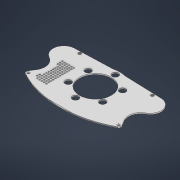
# Autodesk Inventor part: buttonMount-backingPlate
Saved by Autodesk Inventor 2022 (Build 260153000, 153)
## iProperties
Created: 2022-07-18
Part Number: buttonMount-backingPlate
Material: Generic
Document SubType Name: Modeling
Designer: matti
Density: 1 g/cm^3
Appearance: Default
Author: matti
Autodesk Inventor part; units mm, degrees
ref_plane "YZ Plane" through (0, 0, 0) normal (1, 0, 0) x (0, 1, 0)
ref_plane "XZ Plane" through (0, 0, 0) normal (0, 1, 0) x (-1, 0, 0)
ref_plane "XY Plane" through (0, 0, 0) normal (0, 0, 1) x (1, 0, 0)
sketch "Sketch1" plane through (0, 0, 0) normal (0, 1, 0) x (-1, 0, 0)
  arc A0 (1.4897, -42.9742) -> (29.2283, -31.5389) centre (0, 0) ccw
  line L0 (1.4897, -42.9742) -> (76.5814, -40.3711)
  arc A1 (76.5814, -40.3711) -> (86.503, -3.4322) centre (75.8885, -20.3831) ccw
  line L1 (86.503, -3.4322) -> (83.9054, -1.8056)
  arc A2 (77.5688, 25.7598) -> (83.9054, -1.8056) centre (94.5198, 15.1453) ccw
  line L2 (77.5688, 25.7598) -> (83.1923, 34.7403)
  arc A3 (83.1923, 34.7403) -> (84.2595, 38.4553) centre (77.2595, 38.4553) ccw
  line L3 (84.2595, 38.4553) -> (84.2595, 38.4997)
  arc A4 (84.2595, 38.4997) -> (81.6444, 42.8943) centre (79.2595, 38.4997) ccw
  arc A5 (81.6444, 42.8943) -> (0, 63) centre (2.3779, -103.1661) ccw
  arc A6 (0, 63) -> (-81.6444, 42.8943) centre (-2.3779, -103.1661) ccw
  arc A7 (-81.6444, 42.8943) -> (-84.2595, 38.4997) centre (-79.2595, 38.4997) ccw
  line L4 (-84.2595, 38.4997) -> (-84.2595, 38.4553)
  arc A8 (-84.2595, 38.4553) -> (-83.1923, 34.7403) centre (-77.2595, 38.4553) ccw
  line L5 (-83.1923, 34.7403) -> (-77.5688, 25.7598)
  arc A9 (-83.9054, -1.8056) -> (-77.5688, 25.7598) centre (-94.5198, 15.1453) ccw
  line L6 (-83.9054, -1.8056) -> (-86.503, -3.4322)
  arc A10 (-86.503, -3.4322) -> (-76.5814, -40.3711) centre (-75.8885, -20.3831) ccw
  line L7 (-76.5814, -40.3711) -> (-1.4897, -42.9742)
  arc A11 (-29.557, -31.2311) -> (-1.4897, -42.9742) centre (0, 0) ccw
  arc A12 (43, 0) -> (-29.557, -31.2311) centre (0, 0) ccw
  arc A13 (29.2283, -31.5389) -> (43, 0) centre (0, 0) ccw
  arc A14 (43, 0) -> (-33.1962, -27.3316) centre (0, 0) ccw
  arc A15 (13.2392, -24.6723) -> (-13.4968, -24.5323) centre (0, 0) ccw
  circle A16 centre (-30.3109, -17.5) radius 5.5
  circle A17 centre (30.3109, -17.5) radius 5.5
  circle A18 centre (30.3109, 17.5) radius 5.5
  circle A19 centre (0, 35) radius 5.5
  circle A20 centre (-30.3109, 17.5) radius 5.5
  circle A21 centre (0, -35) radius 5.5
  arc A22 (-13.4968, -24.5323) -> (13.2392, -24.6723) centre (0, 0) ccw
  arc A23 (-29.557, -31.2311) -> (-1.4897, -42.9742) centre (0, 0) ccw
  arc A24 (-1.4897, -42.9742) -> (1.4897, -42.9742) centre (0, 0) ccw
  arc A25 (1.4897, -42.9742) -> (29.2283, -31.5389) centre (0, 0) ccw
  arc A26 (32.9081, -27.6777) -> (43, 0) centre (0, 0) ccw
  circle A27 centre (79.2595, 38.4997) radius 0.75
  circle A28 centre (63.8182, -36.3301) radius 1.25
  circle A29 centre (79.2595, 38.4997) radius 1.5
  circle A30 centre (63.8182, -36.3301) radius 2
  arc A31 (0, 61.9999) -> (-81.1674, 42.0154) centre (-2.3779, -103.1661) ccw
  arc A32 (81.1674, 42.0154) -> (0, 61.9999) centre (2.3779, -103.1661) ccw
  arc A33 (83.2595, 38.4997) -> (81.1674, 42.0154) centre (79.2595, 38.4997) ccw
  line L8 (83.2595, 38.4997) -> (83.2595, 38.4553)
  arc A34 (82.3448, 35.271) -> (83.2595, 38.4553) centre (77.2595, 38.4553) ccw
  line L9 (82.3448, 35.271) -> (76.7213, 26.2905)
  arc A35 (76.7213, 26.2905) -> (83.3746, -2.6531) centre (94.5198, 15.1453) ccw
  line L10 (83.3746, -2.6531) -> (85.9722, -4.2797)
  arc A36 (76.5468, -39.3717) -> (85.9722, -4.2797) centre (75.8885, -20.3831) ccw
  line L11 (-10.6691, -41.6554) -> (-76.5468, -39.3717)
  arc A37 (-85.9722, -4.2797) -> (-76.5468, -39.3717) centre (-75.8885, -20.3831) ccw
  line L12 (-85.9722, -4.2797) -> (-83.3746, -2.6531)
  arc A38 (-83.3746, -2.6531) -> (-76.7213, 26.2905) centre (-94.5198, 15.1453) ccw
  line L13 (-76.7213, 26.2905) -> (-82.3448, 35.271)
  arc A39 (-83.2595, 38.4553) -> (-82.3448, 35.271) centre (-77.2595, 38.4553) ccw
  line L14 (-83.2595, 38.4553) -> (-83.2595, 38.4997)
  arc A40 (-81.1674, 42.0154) -> (-83.2595, 38.4997) centre (-79.2595, 38.4997) ccw
  line L15 (76.5468, -39.3717) -> (10.6691, -41.6554)
  line L16 (0, 0) -> (0, 12.9729)
  line L17 (0, 0) -> (12.9729, 0) construction
  circle A41 centre (-79.2595, 38.4997) radius 1.5
  circle A42 centre (-79.2595, 38.4997) radius 0.75
  circle A43 centre (-63.8182, -36.3301) radius 2
  circle A44 centre (-63.8182, -36.3301) radius 1.25
  point P0 (-77.2595, 38.4553)
  point P1 (-1.4897, -42.9742)
  dimension "d0" = 1.5
  dimension "d1" = 2.5
  dimension "d3" = 3
  dimension "d4" = 4
  dimension "d6" = 1
  dimension "d7" = 90
  constraints: 65 point on circle, 45 centre point, 36 end point, 6 coincident, 6 symmetric about line, 1 horizontal, 1 perpendicular, 18 other
  measures "d0" diameter of A27
  measures "d1" diameter of A28
  measures "d3" diameter of A29
  measures "d4" diameter of A30
  measures "d6" radial gap between concentric circles of A6 A31
  measures "d7" angle of L17 L16
extrude "Extrusion1" add sketch "Sketch1" along normal blind 2 contours A24 A11 A12 A13 A0 | A0 A13 A12 A11 L11 A37 L12 A38 L13 A39 L14 A40 A31 A32 A33 L8 A34 L9 A35 L10 A36 L15
chamfer "Chamfer1" distance 0.75 angle 45 4 edges at (80.7595, 2, 38.4997) (65.8182, 2, -36.3301) (-61.8182, 2, -36.3301) (-77.7595, 2, 38.4997)
sketch "Sketch2" plane through (0, 2, 0) normal (0, 1, 0) x (1, 0, 0)
  arc A0 (-39.2332, -48.7478) -> (0.0157, -53.5719) centre (-0.7049, 102.6414) ccw
  line L0 (-43, 8.6615) -> (-61.5767, 28.5094)
  line L1 (-72.4279, 0.8961) -> (-72.4279, -43.1434)
  line L2 (-72.4279, -43.1434) -> (-56.6935, -52.2964)
  arc A1 (-61.5767, 28.5094) -> (-82.4964, 5.3099) centre (-75.8885, 20.3831) ccw
  line L3 (-43, 8.6615) -> (-43, -43.9022)
  arc A2 (57.4373, -52.0723) -> (56.4451, -43.938) centre (55.7026, -48.1562) ccw
  arc A3 (-43, -43.9022) -> (-39.2332, -48.7478) centre (-38, -43.9022) ccw
  line L4 (-72.4279, 0.8961) -> (-82.4964, 5.3099)
  arc A4 (-56.6935, -52.2964) -> (57.4373, -52.0723) centre (0.0404, 116.5749) ccw
  arc A5 (0.0157, -53.5719) -> (56.4451, -43.938) centre (-2.1892, 129.4242) ccw
  circle A6 centre (-75.8885, 20.3831) radius 1.1028
  line L5 (-72.4279, -43.1434) -> (-43, -43.1434)
  line L6 (-72.4279, 0.8961) -> (-52.8672, 19.2039)
  line L7 (-43, -43.1434) -> (-47, -43.1434)
  line L8 (-43, -39.1434) -> (-43, -43.1434)
  circle A7 centre (-47, -39.1434) radius 1.25
  line L9 (-72.4279, -43.1434) -> (-68.4279, -43.1434)
  line L10 (-68.4279, -43.1434) -> (-68.4279, -39.1434)
  line L11 (-68.4279, -39.1434) -> (-72.4279, -39.1434)
  line L12 (-72.4279, -39.1434) -> (-72.4279, -43.1434)
  point P0 (0, 0)
  point P1 (0, 0)
  point P2 (-43, -47.7389)
  point P3 (0, -63)
  dimension "d15" = 2.5
  dimension "d16" = 4
  dimension "d17" = 4
  constraints: 26 end point, 13 point on circle, 9 centre point, 3 perpendicular, 3 point on line, 2 horizontal, 2 parallel, 2 tangent
  measures "d15" diameter of A7
  measures "d16" distance of L11.end L10.end
  measures "d17" distance of L10.end L9.end
extrude "Extrusion2" cut sketch "Sketch2" against normal through all contours A7
pattern_linear "Rectangular Pattern1" count 13 spacing 4 along (0, 0, -1) count 6 spacing 4 along (-1, 0, 0) of "Extrusion2"
sketch "Sketch3" plane through (0, 2, 0) normal (0, 1, 0) x (1, 0, 0)
  arc A0 (-76.7213, -26.2905) -> (-83.3746, 2.6531) centre (-94.5198, -15.1453) ccw projected
  line L0 (-76.7213, -26.2905) -> (-82.3448, -35.271) projected
  arc A1 (-82.3448, -35.271) -> (-83.2595, -38.4553) centre (-77.2595, -38.4553) ccw projected
  arc A2 (-83.2595, -38.4997) -> (-81.1674, -42.0154) centre (-79.2595, -38.4997) ccw projected
  line L1 (-85.9722, 4.2797) -> (-83.3746, 2.6531) projected
  arc A3 (0, -61.9999) -> (81.1674, -42.0154) centre (2.3779, 103.1661) ccw projected
  arc A4 (-81.1674, -42.0154) -> (0, -61.9999) centre (-2.3779, 103.1661) ccw projected
  line L2 (-83.2595, -38.4553) -> (-83.2595, -38.4997) projected
  line L3 (-80.665, 12.7552) -> (-78.0674, 11.1286)
  arc A5 (-68.2458, -31.5977) -> (-78.0674, 11.1286) centre (-94.5198, -15.1453) ccw
  line L4 (-68.2458, -31.5977) -> (-67.4078, -30.2594)
  arc A6 (-64.7334, -38.938) -> (0, -51.9988) centre (-2.3779, 103.1661) ccw
  arc A7 (0, -51.9988) -> (76.3976, -33.2263) centre (2.3779, 103.1661) ccw
  arc A8 (-67.4078, -30.2594) -> (-64.7334, -38.938) centre (-62.3225, -33.4437) ccw
  line L5 (0, -51.9988) -> (0, -61.9999)
  arc A9 (-76.5468, 39.3717) -> (-85.9722, 4.2797) centre (-75.8885, 20.3831) ccw projected
  line L6 (-80.665, 12.7552) -> (-85.9722, 4.2797)
  arc A10 (-64.25, -6.1434) -> (-64, -5.8934) centre (-65, -5.1434) ccw projected
  arc A11 (-64.25, -8.1434) -> (-64, -7.8934) centre (-65, -7.1434) ccw projected
  arc A12 (-64.25, -24.1434) -> (-64, -23.8934) centre (-65, -23.1434) ccw projected
  arc A13 (-64.25, -26.1434) -> (-64, -25.8934) centre (-65, -25.1434) ccw projected
  arc A14 (-66.25, -30.1434) -> (-66, -29.8934) centre (-67, -29.1434) ccw projected
  arc A15 (-66.25, -38.1434) -> (-66, -37.8934) centre (-67, -37.1434) ccw projected
  arc A16 (-65.75, -38.1434) -> (-66, -38.3934) centre (-65, -39.1434) ccw projected
  arc A17 (-66.25, -2.1434) -> (-66, -1.8934) centre (-67, -1.1434) ccw projected
  arc A18 (-81.1674, -42.0154) -> (0, -61.9999) centre (-2.3779, 103.1661) ccw projected
  line L7 (-76.7213, -26.2905) -> (-82.3448, -35.271) projected
  arc A19 (-75.8885, -44.7583) -> (-79.533, -30.7807) centre (-87.5671, -40.3395) ccw
  circle A20 centre (-67, 0.8566) radius 1.25 projected
  circle A21 centre (-67, -3.1434) radius 1.25 projected
  circle A22 centre (-63, -11.1434) radius 1.25 projected
  circle A23 centre (-63, -15.1434) radius 1.25 projected
  circle A24 centre (-63, -19.1434) radius 1.25 projected
  circle A25 centre (-67, -27.1434) radius 1.25 projected
  circle A26 centre (-67, -31.1434) radius 1.25 projected
  circle A27 centre (-67, -35.1434) radius 1.25 projected
  circle A28 centre (-63, -39.1434) radius 1.25 projected
  point P0 (0, 0)
  point P1 (-71.0115, -36.0144)
  point P2 (-63.7685, -39.3575)
  point P3 (-65.8913, -38.267)
  point P4 (-66.1525, -38.0623)
  point P5 (-67.699, -36.1071)
  point P6 (-67.4761, -30.2992)
  point P7 (-66.3463, -28.078)
  point P8 (-65.5777, -26.2519)
  point P9 (-64.7852, -23.912)
  point P10 (-64.9308, -24.3915)
  point P11 (-64.3102, -22.101)
  point P12 (-64.311, -8.1863)
  point P13 (-64.932, -5.8953)
  point P14 (-64.7863, -6.375)
  point P15 (-65.5789, -4.0356)
  point P16 (-67.4779, 0.0117)
  point P17 (-66.3477, -2.2097)
  point P18 (-66.4305, -2.0306)
  point P19 (-65.7971, -3.4832)
  point P20 (-65.7964, -26.8059)
  point P21 (-66.4282, -28.2549)
  dimension "d26" = 10
  dimension "d27" = 6
  constraints: 12 point on circle, 8 end point, 5 centre point, 2 tangent, 1 midpoint, 1 point on line, 1 vertical, 6 other
  measures "d26" radial gap between concentric circles of A0 A5
  measures "d27" radius of A8
extrude "Extrusion3" add sketch "Sketch3" against normal up to surface (2 mm away) contours A0 L1 L6 L3 A5 A20 A21 A22 A23 A24 A25 A26 A8 A27 A6 A28 L5 A4 A19 L0 | A5 A20 | A28 A6 | A21 A5 | A5 A21 | A5 A22 | A27 A8 | A5 A23 | A26 L4 A8 | A5 A24 | A26 A5 | A25 A5 | A5 A25 picked at (-67.8638, 0.411) picked at (-63.2937, -39.8328) picked at (-63.9255, -11.2609) picked at (-68.0292, -35.5174) picked at (-63.7614, -15.1953) picked at (-63.9252, -19.026)
sketch "Sketch4" plane through (0, 0, 0) normal (1, 0, 0) x (0, 1, 0)
  line L0 (0, 61.9999) -> (2, 61.9999) projected
  line L1 (0, 61.9999) -> (1, 61.9999)
  line L2 (1, 61.9999) -> (0, 60.9999)
  line L3 (0, 42.0154) -> (0, 62.017) projected
  line L4 (0, 60.9999) -> (0, 61.9999)
  line L5 (1, 61.9999) -> (1, 65.0761)
  line L6 (2, 61.9999) -> (0, 61.9999)
  line L7 (1, 61.9999) -> (2, 60.9999)
  line L8 (2, 42.0154) -> (2, 62.017)
  point P0 (0, 0)
  dimension "d31" = 1
  dimension "d32" = 45
  constraints: 14 end point, 5 symmetric about line, 2 point on line, 1 midpoint, 1 perpendicular, 1 vertical
  measures "d31" distance of L0.start L1.end
  measures "d32" angle of L1 L2
extrude "Extrusion4" cut sketch "Sketch4" along normal mid plane 100 contours L0 L8 L7
sketch "Sketch5" plane through (0, 0, 61.9999) normal (0, 0, -1) x (-1, 0, 0)
  line L0 (-4.7557, 1) -> (-4.7557, 2) projected
  line L1 (0, 0) -> (-81.1674, 0) projected
  line L2 (-81.1674, 0) -> (-81.1674, 2) projected
  line L3 (0, 2) -> (-4.7557, 2) projected
  line L4 (0, 1) -> (0, 2) projected
  line L5 (0, 0) -> (0, 1) projected
  line L6 (0, 1) -> (0, 2) projected
  line L7 (81.1674, 0) -> (0, 0) projected
  line L8 (0, 0) -> (0, 1) projected
  line L9 (81.1674, 2) -> (20.6805, 2) projected
  line L10 (81.1674, 0) -> (81.1674, 2) projected
  arc A0 (20.6805, 0) -> (4.7557, 1) centre (2.3779, -164.166) ccw projected
  line L11 (4.7557, 1) -> (-4.7557, 1)
  line L12 (4.7557, 1) -> (0, 1) projected
  arc A1 (4.7557, 1) -> (20.6805, 2) centre (2.3779, 166.166) ccw projected
  line L13 (4.7557, 2) -> (0, 2) projected
  line L14 (-20.6805, 2) -> (-81.1674, 2) projected
  arc A2 (-20.6805, 2) -> (-4.7557, 1) centre (-2.3779, 166.166) ccw projected
  line L15 (4.7557, 2) -> (4.7557, 1) projected
  point P0 (0, 0)
  constraints: 2 end point, 1 collinear
split_face "Split1"
sketch "Sketch7" plane through (-20.6805, 2, 60.9999) normal (0, 0.7071068, 0.7071068) x (1, 0, 0)
  ellipse E0 centre (23.0583, 232.1658) end of major axis (23.0583, -1.4384) minor radius 165.1831 (25.4362, -1.4142) -> (41.361, 0) ccw projected
  line L0 (0, 0) -> (41.361, 0) projected
  ellipse E1 centre (18.3026, 232.1658) end of major axis (18.3026, -1.4384) minor radius 165.1831 (0, 0) -> (15.9248, -1.4142) ccw projected
  line L1 (15.9248, -1.4142) -> (20.6805, -1.4142) projected
  line L2 (20.6805, -1.4142) -> (25.4362, -1.4142) projected
  point P0 (20.6805, 41.7192)
  constraints: 2 other
extrude "Extrusion6" cut sketch "Sketch7" along normal blind 5
body "Solid1"
